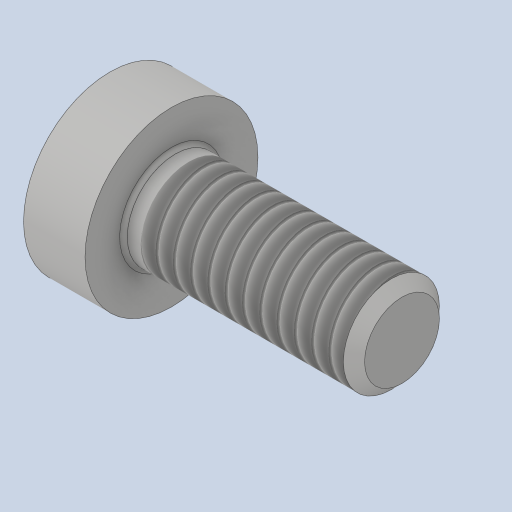
# Autodesk Inventor part: CBSST2_5-6
Saved by Autodesk Inventor 2023 (Build 270158000, 158)
## iProperties
Created: 2024-11-14
Part Number: CBSST2_5-6
Material: Generic
Catalog Web Link: www.cadenas.de
Description: CBS, CBSST-Hexagon Socket Low Head Cap Screws
Vendor: MISUMI
Document SubType Name: Modeling
Designer: psAdmin
Manufacturer: MISUMI
Mass: 0.0519454 g
Surface Area: 1.06719 cm^2
Volume: 0.0519454 cm^3
Density: 1 g/cm^3
Appearance: PSOLRGB-175-175-175
Category: PARTsolutions
Company: MISUMI
PSOL_IDENT_0: {$CADENAS_DATA/23d-libs/misumi/metric/27_screws_nuts/cbsst.prj},171 {VTYP=3D},{NB=CBSST2.5-6},{LINA=
PSOL_IDENT_1: CBSST2.5-6},{NN=CBS, CBSST},{DATE=22.04.2022 09:19:39},{GEOMDATE=16.11.2021 00:42:08},{VERSION=},{LI
PSOL_IDENT_2: NEID=150},{WBVAR=MAT,L},{WBNUMERIC=L}  {NB=CBSST2.5-6},{LINA=CBSST2.5-6},{KT=DUMMY},{PN=CBSST2.5-6},
PSOL_IDENT_3: {MAT=ST},{MATA=  'ST','302HQ Stainless Steel'  },{HARD=-},{ST=-},{SC=A2-50},{M=2.5},{L=6},{LL=Full T
PSOL_IDENT_4: hread},{L1=40},{TYPE=CBS},{M1=2.500},{L0=4,5,6,8,10},{MP=2.5x0.45},{P=0.45},{A=4.5},{E=1.6},{B=1.5},
PSOL_IDENT_5: {TT=1.3},{RR=0.1 or More},{RR1=0.10}
NB: CBSST2.5-6
NN: CBS, CBSST
NT: Hexagon Socket Low Head Cap Screws
NBSYN: $PN.
LINA: CBSST2.5-6
CATALOG: Misumi
PN: CBSST2.5-6
MAT: SUSXM7
HARD: -
ST: -
SC: A2-50
M: 2.5
L: 6
LL: Full Thread
MP: 2.5x0.45
A: 4.5
E: 1.6
B: 1.5
TT: 1.3
RR: 0.1 or More
SUPPLIER: MISUMI
ARTICLENO: CBSST2.5-6
BOMINFO: CBSST2.5-6
CREATOR: CADENAS GmbH
Title: CBSST2.5-6
Author: Cadenas PARTsolutions
Comments: Hexagon Socket Low Head Cap Screws
Autodesk Inventor part; units mm, degrees
sketch "Sketch_1" plane through (0, 0, 0) normal (0, 0, 1) x (1, 0, 0)
  line L0 (6, 0) -> (-1.6, 0)
  line L1 (-1.6, 0) -> (-1.6, 2.25)
  line L2 (-1.6, 2.25) -> (0, 2.25)
  line L3 (0, 2.25) -> (0, 1.35)
  arc A0 (0, 1.35) -> (0.1, 1.25) centre (0.1, 1.35) ccw
  line L4 (0.1, 1.25) -> (5.724, 1.25)
  line L5 (5.724, 1.25) -> (6, 0.974)
  line L6 (6, 0.974) -> (6, 0)
  line L7 (6, 0) -> (-1.6, 0)
  constraints: 16 end point, 2 point on circle, 1 centre point
revolve "Revolution1" add sketch "Sketch_1" angle 360 about axis through (6, 0, 0) along (1, 0, 0)
thread "Thread1" size "M2.5x0.45" class "6g" standard "ISO Metric profile" length 5.274
sketch "Sketch2" plane through (-1.6, 0, 0) normal (-1, 0, 0) x (0, 0, 1)
  point P0 (0, 0)
hole "Hole1" at (-1.6, 0, 0) direction (1, 0, 0) diameter 1.5 depth 1.3 tip angle 140
sketch "Sketch_3" plane through (-1.6, 0, 0) normal (1, 0, 0) x (0, 0, -1)
  line L0 (-0.75, -0.433) -> (0, -0.866)
  line L1 (0, -0.866) -> (0.75, -0.433)
  line L2 (0.75, -0.433) -> (0.75, 0.433)
  line L3 (0.75, 0.433) -> (0, 0.866)
  line L4 (0, 0.866) -> (-0.75, 0.433)
  line L5 (-0.75, 0.433) -> (-0.75, -0.433)
  constraints: 12 end point
extrude "Extrusion1" cut sketch "Sketch_3" along normal blind 1.3
ref_plane "bolt_XY" through (0, 0, 0) normal (1, 0, 0) x (0, 0, -1)
ref_plane "bolt_YZ" through (0, 0, 0) normal (0, 0, -1) x (0, 1, 0)
ref_plane "bolt_ZX" through (0, 0, 0) normal (0, 1, 0) x (1, 0, 0)
ref_plane "bolt_to_nut_XY" through (6, 0, 0) normal (1, 0, 0) x (0, 0, -1)
ref_plane "bolt_to_nut_YZ" through (6, 0, 0) normal (0, 0, -1) x (0, 1, 0)
ref_plane "bolt_to_nut_ZX" through (6, 0, 0) normal (0, 1, 0) x (1, 0, 0)
body "Solid1"
